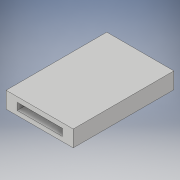
# Autodesk Inventor part: cutter grp 17-2
Saved by Autodesk Inventor 2019 (Build 230136000, 136)
## iProperties
Created: 2020-02-17
Part Number: cutter grp 17-2
Material: Generic
Document SubType Name: Modeling
Designer: Aishwarya
Density: 1 g/cm^3
Appearance: Default
Author: Aishwarya
Autodesk Inventor part; units mm, degrees
ref_plane "YZ Plane" through (0, 0, 0) normal (1, 0, 0) x (0, 1, 0)
ref_plane "XZ Plane" through (0, 0, 0) normal (0, 1, 0) x (-1, 0, 0)
ref_plane "XY Plane" through (0, 0, 0) normal (0, 0, 1) x (1, 0, 0)
sketch "Sketch1" plane through (0, 0, 0) normal (0, 0, 1) x (1, 0, 0)
  line L0 (-5.4331, 6.9327) -> (4.5669, 6.9327)
  line L1 (4.5669, 6.9327) -> (4.5669, 4.4986)
  line L2 (4.5669, 4.4986) -> (-5.4331, 4.4986)
  line L3 (-5.4331, 4.4986) -> (-5.4331, 6.9327)
  point P0 (0, 0)
  dimension "d0" = 10
  constraints: 8 end point, 2 parallel, 1 horizontal, 1 perpendicular
  measures "d0" distance of L1.end L2.end
extrude "Extrusion1" add sketch "Sketch1" along normal blind 15
sketch "Sketch2" plane through (0, 0, 15) normal (0, 0, 1) x (1, 0, 0)
  line L0 (-3.7689, 6.2173) -> (2.9461, 6.2173)
  line L1 (2.9461, 6.2173) -> (2.9461, 5.1689)
  line L2 (2.9461, 5.1689) -> (-3.7689, 5.1689)
  line L3 (-3.7689, 5.1689) -> (-3.7689, 6.2173)
  point P0 (0, 0)
  constraints: 8 end point, 2 parallel, 1 horizontal, 1 perpendicular
extrude "Extrusion2" cut sketch "Sketch2" against normal blind 1.5
body "Solid1"
